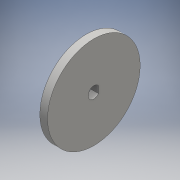
# Autodesk Inventor part: wheel
Saved by Autodesk Inventor 2016 (Build 200138000, 138)
## iProperties
Created: 2015-09-14
Part Number: wheel
Material: Generic
Document SubType Name: Modeling
Designer: Hulbert Office
Density: 1 g/cm^3
Appearance: Default
Author: Hulbert Office
Autodesk Inventor part; units mm, degrees
ref_plane "YZ Plane" through (0, 0, 0) normal (1, 0, 0) x (0, 1, 0)
ref_plane "XZ Plane" through (0, 0, 0) normal (0, 1, 0) x (-1, 0, 0)
ref_plane "XY Plane" through (0, 0, 0) normal (0, 0, 1) x (1, 0, 0)
sketch "Sketch1" plane through (0, 0, 0) normal (1, 0, 0) x (0, 1, 0)
  circle A0 centre (0, 0) radius 24
  circle A1 centre (0, 0) radius 3
  dimension "d0" = 48
  dimension "d1" = 6
  constraints: 2 centre point, 2 coincident
  measures "d0" diameter of A0
  measures "d1" diameter of A1
extrude "Extrusion1" add sketch "Sketch1" along normal blind 4
sketch "Sketch2" plane through (4, 0, 0) normal (1, 0, 0) x (0, 0, -1)
  circle A0 centre (0, 0) radius 3 projected
  line L0 (0, -3) -> (0, 2.4)
  line L1 (0, 2.4) -> (1.8, 2.4)
  line L2 (1.8, 2.4) -> (-1.8, 2.4)
  dimension "d4" = 5.4
  constraints: 6 end point, 3 point on circle, 1 horizontal, 1 perpendicular, 1 vertical
  measures "d4" distance of L0.start L0.end
extrude "Extrusion2" add sketch "Sketch2" against normal blind 4 contours L1 L2 A0
body "Solid1"
